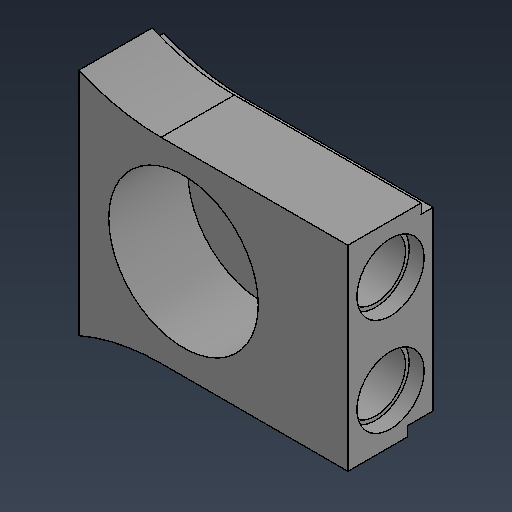
# Autodesk Inventor part: BearigHoldRight
Saved by Autodesk Inventor 2026.2 (Build 302298010, 298A)
## iProperties
Created: 2026-04-04
Part Number: BearigHoldRight
Material: Generic
Document SubType Name: Modeling
Designer: szymo
Density: 1 g/cm^3
Appearance: Default(1)
Author: szymo
Autodesk Inventor part; units mm, degrees
ref_plane "YZ Plane" through (0, 0, 0) normal (1, 0, 0) x (0, 1, 0)
ref_plane "XZ Plane" through (0, 0, 0) normal (0, 1, 0) x (-1, 0, 0)
ref_plane "XY Plane" through (0, 0, 0) normal (0, 0, 1) x (1, 0, 0)
sketch "Sketch1" plane through (0, 0, 0) normal (0, 0, 1) x (1, 0, 0)
  circle A0 centre (-14.5, 55.2958) radius 13.85 projected
  circle A1 centre (-14.5, 55.2958) radius 14.5 projected
  circle A2 centre (-14.5, 14.5) radius 13.85 projected
  circle A3 centre (-14.5, 14.5) radius 14.5 projected
  circle A4 centre (-13, 35.0012) radius 5 projected
  line L0 (0, 65.2958) -> (-20, 65.2958)
  line L1 (-20, 65.2958) -> (-20, -1.7042)
  line L2 (-20, -1.7042) -> (0, -1.7042)
  line L3 (0, -1.7042) -> (0, 65.2958)
  line L4 (-2, 65.2958) -> (-2, -1.7042)
  line L5 (-14.5, 41.4458) -> (-2, 41.4458)
  line L6 (-14.5, 40.7958) -> (-2, 40.7958)
  line L7 (-14.5, 28.35) -> (-2, 28.35)
  line L8 (-14.5, 29) -> (-2, 29)
  point P0 (0, 0)
  point P1 (-20, 42.5847)
  point P2 (-20, 27.2111)
  point P3 (-20, 27.9164)
  point P4 (-20, 41.8794)
  dimension "d0" = 67
  dimension "d1" = 2
  dimension "d2" = 2
  constraints: 18 end point, 6 perpendicular, 6 point on line, 5 horizontal, 2 parallel, 9 other
  measures "d0" distance of L2.end L0.start
  measures "d1" distance edge to line of A4 L1
  measures "d2" distance between parallel lines of L3 L4
ref_plane "Work Plane1" through (-33.5144, -4.5144, -4) normal (0, 0, 1) x (0.9204317, 0.3909035, 0)
extrude "Extrusion1" add sketch "Sketch1" against normal up to surface (4 mm away) contours L5 A1 L1 A0 | L5 L4 L6 A1 | A1 L6 L4 L8 A3 L1 | A3 L7 A2 L1 | L4 L7 A3 L8
ref_plane "Work Plane2" through (-34.9799, 34.8159, -4.9) normal (0, 0, 1) x (0.7419326, 0.6704745, 0)
extrude "Extrusion2" add sketch "Sketch1" against normal up to surface (4.9 mm away) contours L5 A1 L1 A0 | L5 L4 L6 A1 | A1 L6 L4 L8 A3 L1
extrude "Extrusion3" add sketch "Sketch1" against normal blind 5.3 contours A1 L6 L4 L8 A3 L1
sketch "Sketch2" plane through (0, 0, -5.3) normal (0, 0, -1) x (-1, 0, 0)
  line L0 (2, 40.7958) -> (2, 29) projected
  line L1 (2, 29) -> (14.5, 29) projected
  arc A0 (20, 27.9164) -> (14.5, 29) centre (14.5, 14.5) ccw projected
  line L2 (20, 27.9164) -> (20, 41.8794) projected
  arc A1 (14.5, 40.7958) -> (20, 41.8794) centre (14.5, 55.2958) ccw projected
  line L3 (14.5, 40.7958) -> (2, 40.7958) projected
  circle A2 centre (13, 35.0012) radius 5 projected
  point P0 (0, 0)
extrude "Extrusion4" add sketch "Sketch2" along normal blind 0.4 contours L3 A1 L2 A0 L1 L0 | A2
sketch "Sketch3" plane through (-2, 28.35, 0) normal (1, 0, 0) x (0, 0, -1)
  line L0 (4.9, 13.0958) -> (4.9, 12.4458) projected
  line L1 (0, 13.0958) -> (4.9, 13.0958) projected
  line L2 (0, 0) -> (0, 13.0958) projected
  line L3 (0, 0) -> (4, 0) projected
  line L4 (4, 0.65) -> (4, 0) projected
  line L5 (4, 0.65) -> (5.7, 0.65) projected
  line L6 (5.7, 12.4458) -> (5.7, 0.65) projected
  line L7 (4.9, 12.4458) -> (5.7, 12.4458) projected
  line L8 (0, 6.5479) -> (5.7, 6.5479)
  line L9 (5.7, -0.4336) -> (5.7, 13.5294) projected
  line L10 (0, 13.0958) -> (5.7, 6.5479)
  line L11 (5.7, 6.5479) -> (0, 0)
  line L12 (0, 6.5479) -> (2.85, 3.274)
  line L13 (0, 6.5479) -> (2.85, 9.8219)
  point P0 (0, -28.35)
  dimension "d11" = 6.5479
  dimension "d12" = 6.5479
  constraints: 10 end point, 4 midpoint, 2 coincident, 1 perpendicular
  measures "d11" distance between parallel lines of L1 L8
  measures "d12" distance between parallel lines of L3 L8
hole "Hole1" at (-2, 38.1719, -2.85) at (-2, 31.624, -2.85) direction (-1, 0, 0) diameter 4 depth 5.5 counterbore diameter 4.5 counterbore depth 1
equation "\"d11\" = d12"
body "Solid1"
